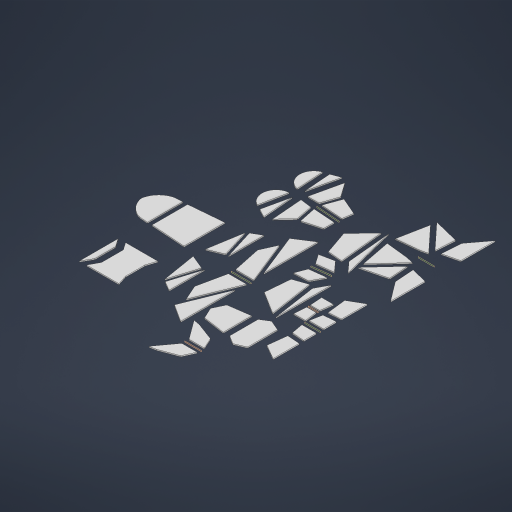
# Autodesk Inventor part: CabezaGodzillaPlanchado
Saved by Autodesk Inventor 2024 (Build 280153000, 153)
## iProperties
Created: 2024-04-16
Part Number: CabezaGodzillaPlanchado
Material: Genérico
Document SubType Name: Modeling
Designer: nicol
Density: 1 g/cm^3
Appearance: Valor por defecto
Author: nicol
Autodesk Inventor part; units mm, degrees
ref_plane "YZ Plane" through (0, 0, 0) normal (1, 0, 0) x (0, 1, 0)
ref_plane "XZ Plane" through (0, 0, 0) normal (0, 1, 0) x (-1, 0, 0)
ref_plane "XY Plane" through (0, 0, 0) normal (0, 0, 1) x (1, 0, 0)
sketch "Boceto1" plane through (0, 0, 0) normal (0, 1, 0) x (-1, 0, 0)
  line L0 (-29.3167, -66.9574) -> (-2.3167, -66.9574) construction
  line L1 (-29.3167, 40.2679) -> (-2.3167, 40.2679) construction
  line L2 (-6.4194, -52.6496) -> (53.9869, -44.16)
  line L3 (-6.4194, -52.6496) -> (54.5806, -52.6496) construction
  line L4 (-6.4194, 25.9601) -> (53.9869, 17.4705)
  line L5 (-6.4194, 25.9601) -> (54.5806, 25.9601) construction
  line L6 (53.9869, -44.16) -> (53.9869, 17.4705)
  line L7 (68.3563, -13.3448) -> (53.9869, -44.16)
  line L8 (68.3563, -13.3448) -> (53.9869, 17.4705)
  line L9 (-6.4194, 25.9601) -> (-6.4194, -52.6496)
  point P0 (0, 0)
  dimension "d4" = 27
  dimension "d6" = 27
  dimension "d8" = 61
  dimension "d9" = 8
  dimension "d10" = 61
  dimension "d11" = 8
  dimension "d12" = 123
  constraints: 20 end point, 4 horizontal, 2 equal length, 1 vertical
  measures "d4" distance of L0.start L2.start
  measures "d6" distance of L1.start L4.start
  measures "d8" distance of L2.start L2.end
  measures "d9" angle of L3 L2
  measures "d10" distance of L4.start L4.end
  measures "d11" angle of L4 L5
  measures "d12" angle of L2 L7
extrude "Extrusión1" add sketch "Boceto1" along normal blind 3
sketch "Boceto3" plane through (0, 0, 0) normal (0, 1, 0) x (-1, 0, 0)
  line L0 (-75.4701, 27.9457) -> (-75.4701, -55.0543)
  line L1 (-75.4701, -55.0543) -> (-46.9345, -67.167)
  line L2 (-75.4701, 27.9457) -> (-46.9345, 40.0583)
  line L3 (-46.9345, 40.0583) -> (-46.9345, -67.167)
  line L4 (-46.9345, -67.167) -> (-24.0372, -52.8592)
  line L5 (-46.9345, 40.0583) -> (-24.0372, 25.7505)
  line L6 (-24.0372, 25.7505) -> (-24.0372, -52.8592)
  point P0 (0, 0)
  dimension "d23" = 83
  dimension "d24" = 31
  dimension "d25" = 113
  dimension "d26" = 31
  dimension "d27" = 27
  dimension "d28" = 27
  constraints: 14 end point, 2 vertical
  measures "d23" distance of L0.start L0.end
  measures "d24" distance of L0.end L1.end
  measures "d25" angle of L1 L0
  measures "d26" distance of L0.start L3.start
  measures "d27" distance of L1.end L4.end
  measures "d28" distance of L3.start L6.start
extrude "Extrusión2" add sketch "Boceto3" along normal blind 3 separate body
sketch "Boceto4" plane through (0, 0, 0) normal (0, 1, 0) x (-1, 0, 0)
  line L0 (32.6665, -126.7711) -> (26.6898, -195.0845)
  line L1 (-29.245, -88.0845) -> (32.6665, -126.7711)
  line L2 (-29.245, -88.0845) -> (-11.0895, -208.2269)
  line L3 (-11.0895, -208.2269) -> (26.6898, -195.0845)
  point P0 (0, 0)
  point P1 (-26.85, -250.6205)
  point P2 (-29.245, -165.0845)
  dimension "d51" = 117
  dimension "d52" = 40
  constraints: 8 end point, 2 other
  measures "d51" angle of L0 L1
  measures "d52" distance of L2.end L0.end
extrude "Extrusión3" add sketch "Boceto4" along normal blind 3 separate body
sketch "Boceto5" plane through (0, 0, 0) normal (0, 1, 0) x (-1, 0, 0)
  line L0 (-43.1322, -82.572) -> (-43.1322, -236.572)
  line L1 (-24.9767, -202.7144) -> (-43.1322, -236.572)
  line L2 (-43.1322, -82.572) -> (-24.9767, -202.7144)
  point P0 (0, 0)
  point P1 (-43.1322, -159.572)
  dimension "d55" = 154
  constraints: 6 end point, 1 midpoint, 1 vertical, 1 other
  measures "d55" distance of L0.start L0.end
extrude "Extrusión4" add sketch "Boceto5" along normal blind 3 separate body
sketch "Boceto6" plane through (0, 0, 0) normal (0, 1, 0) x (-1, 0, 0)
  line L0 (-19.3821, -249.0178) -> (27.2676, -243.2899)
  line L1 (27.2676, -243.2899) -> (38.7354, -213.4154)
  line L2 (38.7354, -213.4154) -> (-1.2265, -215.1601)
  line L3 (-1.2265, -215.1601) -> (-19.3821, -249.0178)
  point P0 (0, 0)
  dimension "d58" = 47
  dimension "d59" = 32
  dimension "d60" = 40
  dimension "d61" = 118
  dimension "d62" = 66.5
  dimension "d63" = 120.702
  constraints: 8 end point
  measures "d58" distance of L0.start L0.end
  measures "d59" distance of L0.end L2.start
  measures "d60" distance of L2.start L3.start
  measures "d61" angle of L0 L1
  measures "d62" angle of L1 L2
  measures "d63" angle of L3 L2
extrude "Extrusión5" add sketch "Boceto6" along normal blind 3 separate body
ref_plane "Plano de trabajo1" through (-28.6691, 0, -254.7042) normal (-0.1219, 0, -0.9925) x (-0.9925, 0, 0.1219)
mirror "Simetría1" about plane through (-28.6691, 0, -254.7042) normal (-0.1219, 0, -0.9925) bodies 3 5 4
sketch "Boceto7" plane through (0, 0, 0) normal (0, 1, 0) x (-1, 0, 0)
  line L0 (-137.4518, -100.7221) -> (-97.4518, -100.7221)
  line L1 (-97.4518, -100.7221) -> (-103.5489, -68.2902)
  line L2 (-103.5489, -68.2902) -> (-137.4518, -65.7221)
  line L3 (-137.4518, -65.7221) -> (-137.4518, -100.7221)
  point P0 (0, 0)
  dimension "d67" = 40
  dimension "d68" = 33
  dimension "d69" = 34
  dimension "d70" = 35
  constraints: 8 end point
  measures "d67" distance of L3.end L1.start
  measures "d68" distance of L1.start L2.start
  measures "d69" distance of L2.start L3.start
  measures "d70" distance of L3.end L3.start
extrude "Extrusión6" add sketch "Boceto7" along normal blind 3 separate body
sketch "Boceto8" plane through (0, 0, 0) normal (0, 1, 0) x (-1, 0, 0)
  line L0 (-138.3377, 19.8369) -> (-138.3377, -52.1631)
  line L1 (-104.4348, -54.7313) -> (-138.3377, -52.1631)
  line L2 (-104.4348, -54.7313) -> (-98.4508, -3.0767)
  line L3 (-98.4508, -3.0767) -> (-138.3377, 19.8369)
  point P0 (0, 0)
  dimension "d73" = 34
  dimension "d74" = 52
  dimension "d75" = 46
  constraints: 8 end point, 1 vertical
  measures "d73" distance of L2.start L0.end
  measures "d74" distance of L2.start L3.start
  measures "d75" distance of L3.start L3.end
extrude "Extrusión7" add sketch "Boceto8" along normal blind 3 separate body
ref_plane "Plano de trabajo2" through (137.4518, 0, -110.7221) normal (0, 0, -1) x (-1, 0, 0)
mirror "Simetría2" about plane through (137.4518, 0, -110.7221) normal (0, 0, -1) bodies 7 6
sketch "Boceto9" plane through (0, 0, 0) normal (0, 1, 0) x (-1, 0, 0)
  line L0 (76.7272, -121.4273) -> (126.7272, -121.4273)
  line L1 (126.7272, -121.4273) -> (143.1522, -44.1536)
  line L2 (143.1522, -44.1536) -> (124.4423, -2.1306)
  line L3 (124.4423, -2.1306) -> (76.7272, -121.4273)
  point P0 (0, 0)
  dimension "d84" = 50
  dimension "d85" = 79
  dimension "d86" = 102
  dimension "d87" = 46
  dimension "d88" = 144
  constraints: 8 end point
  measures "d84" distance of L3.end L1.start
  measures "d85" distance of L1.start L2.start
  measures "d86" angle of L1 L0
  measures "d87" distance of L2.start L3.start
  measures "d88" angle of L2 L1
extrude "Extrusión8" add sketch "Boceto9" along normal blind 3 separate body
sketch "Boceto10" plane through (0, 0, 0) normal (0, 1, 0) x (-1, 0, 0)
  line L0 (79.0325, 58.7177) -> (79.0325, -91.2823)
  line L1 (126.7476, 28.0144) -> (79.0325, 58.7177)
  line L2 (126.7476, 28.0144) -> (79.0325, -91.2823)
  point P0 (0, 0)
  dimension "d91" = 150
  constraints: 6 end point, 1 vertical
  measures "d91" distance of L0.start L0.end
extrude "Extrusión9" add sketch "Boceto10" along normal blind 3 separate body
ref_plane "Plano de trabajo3" through (-76.7272, 0, -131.4273) normal (0, 0, -1) x (-1, 0, 0)
mirror "Simetría3" about plane through (-76.7272, 0, -131.4273) normal (0, 0, -1) bodies 9 8
sketch "Boceto11" plane through (0, 0, 0) normal (0, 1, 0) x (-1, 0, 0)
  line L0 (62.604, 37.8442) -> (24.1836, 90.2739)
  line L1 (-3.8016, 59.3352) -> (44.9054, 41.1244)
  line L2 (24.1836, 90.2739) -> (-17.9012, 90.2739)
  line L3 (-17.9012, 90.2739) -> (-3.8016, 59.3352)
  line L4 (62.604, 37.8442) -> (44.9054, 41.1244)
  point P0 (0, 0)
  dimension "d101" = 34
  dimension "d102" = 52
  dimension "d103" = 135
  dimension "d104" = 18
  dimension "d105" = 65
  constraints: 10 end point, 1 horizontal
  measures "d101" distance of L2.end L1.start
  measures "d102" distance of L1.start L1.end
  measures "d103" angle of L1 L3
  measures "d104" distance of L1.end L0.start
  measures "d105" distance of L0.start L2.start
extrude "Extrusión10" add sketch "Boceto11" along normal blind 3 separate body
ref_plane "Plano de trabajo4" through (-24.1836, 0, 100.2739) normal (0, 0, 1) x (1, 0, 0)
mirror "Simetría4" about plane through (-24.1836, 0, 100.2739) normal (0, 0, 1) bodies 10
sketch "Boceto12" plane through (0, 0, 0) normal (0, 1, 0) x (-1, 0, 0)
  line L0 (-143.438, -280.8968) -> (-143.438, -375.8968)
  line L1 (-143.438, -280.8968) -> (-103.7182, -333.6067)
  line L2 (-103.7182, -333.6067) -> (-100.0211, -386.4776)
  line L3 (-100.0211, -386.4776) -> (-143.438, -375.8968)
  point P0 (0, 0)
  dimension "d109" = 95
  dimension "d110" = 66
  dimension "d111" = 53
  constraints: 8 end point, 1 vertical
  measures "d109" distance of L0.start L3.end
  measures "d110" distance of L0.start L1.end
  measures "d111" distance of L1.end L3.start
extrude "Extrusión11" add sketch "Boceto12" along normal blind 3 separate body
sketch "Boceto13" plane through (0, 0, 0) normal (0, 1, 0) x (-1, 0, 0)
  line L0 (-107.2749, -334.1906) -> (-38.3839, -317.0141)
  line L1 (-107.2749, -334.1906) -> (-103.5778, -387.0614)
  line L2 (-103.5778, -387.0614) -> (-38.3839, -317.0141)
  point P0 (0, 0)
  dimension "d114" = 71
  dimension "d115" = 53
  dimension "d116" = 100
  constraints: 6 end point
  measures "d114" distance of L0.start L0.end
  measures "d115" distance of L0.start L1.end
  measures "d116" angle of L0 L1
move or copy body "Desplazar cuerpo1" bodies to move or copy 11 copy no translate (20, 0, 0)
extrude "Extrusión12" add sketch "Boceto13" along normal blind 3 separate body
sketch "Boceto14" plane through (0, 0, 0) normal (0, 1, 0) x (-1, 0, 0)
  line L0 (-36.368, -332.7728) -> (-20.5309, -414.2478)
  line L1 (-101.5619, -402.8201) -> (-36.368, -332.7728)
  line L2 (-101.5619, -402.8201) -> (-82.1306, -407.5556)
  line L3 (-82.1306, -407.5556) -> (-20.5309, -414.2478)
  point P0 (0, 0)
  dimension "d122" = 83
  dimension "d123" = 20
  constraints: 8 end point
  measures "d122" distance of L1.end L3.end
  measures "d123" distance of L2.start L3.start
extrude "Extrusión13" add sketch "Boceto14" along normal blind 3 separate body
ref_plane "Plano de trabajo5" through (137.4518, 0, -425.4721) normal (0, 0, -1) x (-1, 0, 0)
mirror "Simetría5" about plane through (137.4518, 0, -425.4721) normal (0, 0, -1) bodies 11 12 13
sketch "Boceto15" plane through (0, 0, 0) normal (0, 1, 0) x (-1, 0, 0)
  line L0 (169.74, 0) -> (169.74, -98)
  line L1 (169.74, -98) -> (195.1764, -14.8015)
  line L2 (195.1764, -14.8015) -> (169.74, 0)
  line L3 (169.74, 0) -> (195.1764, -14.8015)
  line L4 (195.1764, -14.8015) -> (169.74, -98)
  point P0 (0, 0)
  constraints: 10 end point, 2 collinear, 1 vertical
extrude "Extrusión14" add sketch "Boceto15" along normal blind 3 separate body
sketch "Boceto16" plane through (0, 0, 0) normal (0, 1, 0) x (-1, 0, 0)
  line L0 (177.8383, -97.9662) -> (217.5248, -114.5186)
  line L1 (217.5248, -114.5186) -> (202.0742, -20.7834)
  line L2 (202.0742, -20.7834) -> (177.8383, -97.9662)
  point P0 (0, 0)
  constraints: 6 end point
extrude "Extrusión15" add sketch "Boceto16" along normal blind 3 separate body
mirror "Simetría6" about plane through (-76.7272, 0, -131.4273) normal (0, 0, -1) bodies 15 14
sketch "Boceto17" plane through (0, 0, 0) normal (0, 1, 0) x (-1, 0, 0)
  line L0 (263.6751, 0) -> (263.6751, -27)
  line L1 (263.6751, -27) -> (255.0226, -53.6296)
  line L2 (255.0226, -53.6296) -> (344.0226, -53.6296)
  line L3 (344.0226, -53.6296) -> (329.6832, -33.1508)
  line L4 (329.6832, -33.1508) -> (329.6832, 27.3492)
  line L5 (263.6751, 0) -> (263.6751, 27.3492)
  line L6 (263.6751, 27.3492) -> (255.0226, 53.9788)
  line L7 (255.0226, 53.9788) -> (344.0226, 53.9788)
  line L8 (344.0226, 53.9788) -> (329.6832, 27.3492)
  point P0 (0, 0)
  constraints: 18 end point, 2 perpendicular, 2 vertical, 1 horizontal
extrude "Extrusión16" add sketch "Boceto17" along normal blind 3 separate body
sketch "Boceto18" plane through (0, 0, 0) normal (0, 1, 0) x (-1, 0, 0)
  line L0 (348.3037, 0) -> (348.3037, -30.25)
  line L1 (348.3037, -30.25) -> (363.8051, -52.3883)
  line L2 (344.0226, -53.6296) -> (329.6832, -33.1508) projected
  line L3 (363.8051, -52.3883) -> (363.8051, 53.9788)
  line L4 (363.8051, 53.9788) -> (348.3037, 27.3492)
  line L5 (348.3037, 27.3492) -> (348.3037, 0)
  point P0 (0, 0)
  constraints: 10 end point, 2 parallel, 1 collinear, 1 point on line, 1 vertical
extrude "Extrusión17" add sketch "Boceto18" along normal blind 3 separate body
sketch "Boceto19" plane through (0, 0, 0) normal (0, 1, 0) x (-1, 0, 0)
  line L0 (255.0226, -126.415) -> (255.0226, -239.415)
  line L1 (255.0226, -239.415) -> (349.6611, -231.1352)
  line L2 (349.6611, -231.1352) -> (349.6611, -132.8352)
  line L3 (349.6611, -132.8352) -> (255.0226, -126.415)
  line L4 (349.6611, -181.9852) -> (283.6611, -181.9852)
  line L5 (283.6611, -181.9852) -> (349.6611, -132.8352)
  line L6 (283.6611, -181.9852) -> (349.6611, -231.1352)
  point P0 (0, 0)
  constraints: 14 end point, 2 vertical, 1 horizontal, 1 midpoint
extrude "Extrusión18" add sketch "Boceto19" along normal blind 3 separate body
sketch "Boceto20" plane through (0, 0, 0) normal (0, 1, 0) x (-1, 0, 0)
  line L0 (362.7, -132.8352) -> (362.7, -231.1352)
  line L1 (362.7, -231.1352) -> (386.6087, -229.0435)
  line L2 (362.7, -132.8352) -> (386.6087, -134.8847)
  line L3 (362.7, -181.9852) -> (428.7, -181.9852)
  arc A0 (386.6087, -229.0435) -> (428.7, -181.9852) centre (370.7228, -172.4808) ccw
  arc A1 (428.7, -181.9852) -> (386.6087, -134.9269) centre (370.7228, -191.4896) ccw
  line L4 (386.6087, -134.9269) -> (386.6087, -134.8847)
  point P0 (0, 0)
  constraints: 10 end point, 4 point on circle, 2 centre point, 2 symmetric about line, 2 vertical, 1 horizontal, 1 midpoint, 1 other
extrude "Extrusión19" add sketch "Boceto20" along normal blind 3 separate body
sketch "Boceto21" plane through (0, 0, 0) normal (0, 1, 0) x (-1, 0, 0)
  line L0 (103.5512, -362.2279) -> (103.5512, -391.2279)
  line L1 (103.5512, -391.2279) -> (163.405, -395.4133)
  line L2 (163.405, -395.4133) -> (153.4253, -348.4622)
  line L3 (153.4253, -348.4622) -> (103.5512, -362.2279)
  line L4 (171.6428, -395.9894) -> (164.9218, -348.4622)
  line L5 (164.9218, -348.4622) -> (198.9298, -313.1854)
  line L6 (198.9298, -313.1854) -> (205.1223, -400.6653)
  line L7 (205.1223, -400.6653) -> (171.6428, -395.9894)
  point P0 (0, 0)
  dimension "d139" = 74
  dimension "d140" = 128
  dimension "d141" = 48
  dimension "d142" = 78
  dimension "d143" = 106
  constraints: 16 end point, 1 vertical
  measures "d139" angle of L1 L2
  measures "d140" angle of L5 L4
  measures "d141" angle of L6 L5
  measures "d142" angle of L6 L7
  measures "d143" angle of L4 L7
extrude "Extrusión20" add sketch "Boceto21" along normal blind 3 separate body contours L3 L2 L1 L0
sketch "Boceto22" plane through (0, 0, 0) normal (0, 1, 0) x (-1, 0, 0)
  line L0 (163.7555, -348.7087) -> (196.6786, -313.7792)
  line L1 (196.6786, -313.7792) -> (203.7161, -399.4907)
  line L2 (203.7161, -399.4907) -> (172.5917, -395.5002)
  line L3 (172.5917, -395.5002) -> (163.7555, -348.7087)
  point P0 (0, 0)
  point P1 (-131.9969, 899.7506)
  dimension "d152" = 86
  dimension "d153" = 48
  dimension "d154" = 78
  constraints: 8 end point
  measures "d152" distance of L0.end L1.end
  measures "d153" angle of L1 L0
  measures "d154" angle of L2 L1
extrude "Extrusión21" add sketch "Boceto22" along normal blind 3 separate body
sketch "Boceto23" plane through (0, 0, 0) normal (0, 1, 0) x (-1, 0, 0)
  line L0 (214.9004, -307.4344) -> (221.8656, -393.1519)
  line L1 (221.8656, -393.1519) -> (237.9126, -319.8887)
  line L2 (237.9126, -319.8887) -> (214.9004, -307.4344)
  point P0 (0, 0)
  dimension "d157" = 86
  dimension "d158" = 75
  dimension "d159" = 17
  constraints: 6 end point
  measures "d157" distance of L0.start L0.end
  measures "d158" distance of L0.end L1.end
  measures "d159" angle of L1 L0
extrude "Extrusión22" add sketch "Boceto23" along normal blind 3 separate body
sketch "Boceto24" plane through (0, 0, 0) normal (0, 1, 0) x (-1, 0, 0)
  line L0 (252.4422, -326.8093) -> (237.2186, -400.248)
  line L1 (237.2186, -400.248) -> (242.6991, -373.81)
  line L2 (242.6991, -373.81) -> (269.137, -379.2905)
  arc A0 (237.2186, -400.248) -> (252.4422, -326.8093) centre (234.5489, -361.3973) ccw
  point P0 (0, 0)
  dimension "d162" = 75
  dimension "d163" = 27
  dimension "d164" = 27
  dimension "d165" = 90
  constraints: 6 end point, 3 point on circle, 1 centre point, 1 perpendicular, 1 point on line
  measures "d162" distance of L0.start L0.end
  measures "d163" distance of L0.end L1.end
  measures "d164" distance of L1.end L2.end
  measures "d165" angle of L1 L2
extrude "Extrusión23" add sketch "Boceto24" along normal blind 3 separate body
ref_plane "Plano de trabajo6" through (-162.7075, 0, -405.389) normal (0.0698, 0, -0.9976) x (-0.9976, 0, -0.0698)
mirror "Simetría7" about plane through (-162.7075, 0, -405.389) normal (0.0698, 0, -0.9976) bodies 20 21 22 23
sketch "Boceto25" plane through (0, 0, 0) normal (0, 1, 0) x (-1, 0, 0)
  line L0 (-87.7951, -159.7077) -> (-92.233, -193.4168)
  line L1 (-87.7951, -159.7077) -> (-53.7951, -159.7077) construction
  line L2 (-92.233, -193.4168) -> (-62.233, -193.4168)
  line L3 (-87.7951, -159.7077) -> (-61.7951, -159.7077)
  line L4 (-61.7951, -159.7077) -> (-59.4379, -193.4168)
  line L5 (-59.4379, -193.4168) -> (-92.233, -193.4168)
  point P0 (0, 0)
  dimension "d169" = 34
  dimension "d170" = 97.5
  dimension "d171" = 30
  dimension "d172" = 26
  dimension "d173" = 94
  constraints: 12 end point, 2 horizontal, 2 point on line, 1 equal length, 1 parallel
  measures "d169" distance of L0.start L0.end
  measures "d170" angle of L0 L1
  measures "d171" distance of L0.end L2.end
  measures "d172" distance of L0.start L3.end
  measures "d173" angle of L3 L4
extrude "Extrusión24" add sketch "Boceto25" along normal blind 3 separate body
ref_plane "Plano de trabajo7" through (61.7951, 0, -154.7077) normal (0, 0, 1) x (1, 0, 0)
mirror "Simetría8" about plane through (61.7951, 0, -154.7077) normal (0, 0, 1) bodies 24
